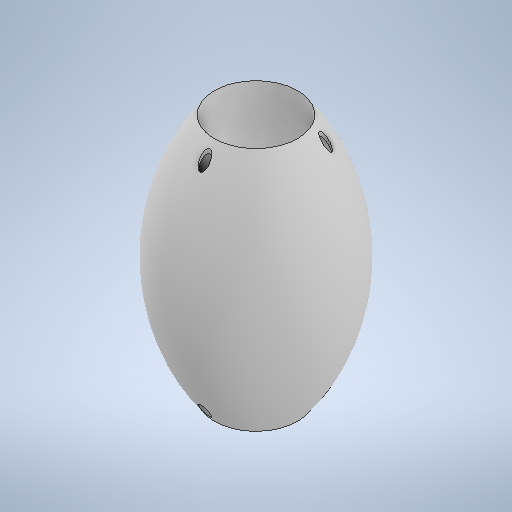
# Autodesk Inventor part: Buoy 8 TallSkinnySphere
Saved by Autodesk Inventor 2025 (Build 290162000, 162)
## iProperties
Created: 2024-07-03
Part Number: Buoy 8 TallSkinnySphere
Material: Generic
Document SubType Name: Modeling
Designer: track
Density: 1 g/cm^3
Appearance: Default
Author: track
Autodesk Inventor part; units mm, degrees
ref_plane "YZ Plane" through (0, 0, 0) normal (1, 0, 0) x (0, 1, 0)
ref_plane "XZ Plane" through (0, 0, 0) normal (0, 1, 0) x (-1, 0, 0)
ref_plane "XY Plane" through (0, 0, 0) normal (0, 0, 1) x (1, 0, 0)
sketch "Sketch1" plane through (0, 0, 0) normal (0, 0, 1) x (1, 0, 0)
  line L0 (0, 0) -> (0, 152.4) construction
  line L1 (25.9, 0) -> (25.9, 152.4)
  line L2 (0, 0) -> (25.9, 0) construction
  arc A0 (25.9, 0) -> (25.9, 152.4) centre (-75.7, 76.2) ccw
  line L3 (27.4, 147.7586) -> (27.4, 4.6414)
  arc A1 (27.4, 4.6414) -> (27.4, 147.7586) centre (-75.7, 76.2) ccw
  point P0 (51.3, 76.2)
  dimension "d0" = 152.4
  dimension "d1" = 25.9
  dimension "d2" = 25.4
  dimension "d3" = 1.5
  constraints: 8 end point, 5 point on circle, 2 centre point, 2 vertical, 1 horizontal, 1 other
  measures "d0" distance of L1.start L1.end
  measures "d1" distance of L0.start L1.start
  measures "d2" distance from line of L1 point (51.3, 76.2)
  measures "d3" distance between parallel lines of L1 L3
revolve "Revolution1" add sketch "Sketch1" angle 360 about axis through (0, 0, 0) along (0, 1, 0)
sketch "Sketch2" plane through (0, 0, 0) normal (0, 1, 0) x (-1, 0, 0)
  circle A0 centre (0, 0) radius 27.4 projected
  line L0 (0, 0) -> (0, 31.75)
  circle A1 centre (0, 31.75) radius 3
  dimension "d5" = 6
  dimension "d6" = 31.75
  constraints: 2 end point, 1 centre point, 1 coincident, 1 vertical
  measures "d5" diameter of A1
  measures "d6" distance of L0.start L0.end
extrude "Extrusion1" cut sketch "Sketch2" along normal through all contours A1
pattern_circular "Circular Pattern1" count 3 over 360 about axis through (0, 76.2, 0) along (0, 1, 0) of "Extrusion1"
body "Solid1"
